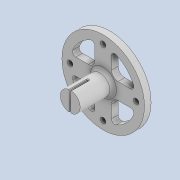
# Autodesk Inventor part: tendon_wh_1_mod
Saved by Autodesk Inventor 2020 (Build 240168000, 168)
## iProperties
Created: 2020-12-06
Part Number: tendon_wh_1_mod
Material: Generic
Document SubType Name: Modeling
Designer: Shuang Peng
Density: 1 g/cm^3
Appearance: Default
Author: Shuang Peng
Autodesk Inventor part; units mm, degrees
ref_plane "YZ Plane" through (0, 0, 0) normal (1, 0, 0) x (0, 1, 0)
ref_plane "XZ Plane" through (0, 0, 0) normal (0, 1, 0) x (-1, 0, 0)
ref_plane "XY Plane" through (0, 0, 0) normal (0, 0, 1) x (1, 0, 0)
sketch "Sketch1" plane through (0, 0, 0) normal (0, 0, 1) x (1, 0, 0)
  circle A0 centre (-10, 0) radius 1 projected
  circle A1 centre (0, 10) radius 1 projected
  circle A2 centre (0, -10) radius 1 projected
  circle A3 centre (10, 0) radius 1 projected
  circle A4 centre (0, 0) radius 1.5 projected
  arc A5 (10.8355, 3.8525) -> (3.8525, 10.8355) centre (0, 0) ccw projected
  arc A6 (9.4222, 1.85) -> (10.8355, 3.8525) centre (9.4222, 3.35) ccw projected
  line L0 (9.4222, 1.85) -> (3.35, 1.85) projected
  arc A7 (1.85, 3.35) -> (3.35, 1.85) centre (3.35, 3.35) ccw projected
  line L1 (1.85, 3.35) -> (1.85, 9.4222) projected
  arc A8 (3.8525, 10.8355) -> (1.85, 9.4222) centre (3.35, 9.4222) ccw projected
  line L2 (-1.85, 9.4222) -> (-1.85, 3.35) projected
  arc A9 (-3.35, 1.85) -> (-1.85, 3.35) centre (-3.35, 3.35) ccw projected
  line L3 (-3.35, 1.85) -> (-9.4222, 1.85) projected
  arc A10 (-10.8355, 3.8525) -> (-9.4222, 1.85) centre (-9.4222, 3.35) ccw projected
  arc A11 (-3.8525, 10.8355) -> (-10.8355, 3.8525) centre (0, 0) ccw projected
  arc A12 (-1.85, 9.4222) -> (-3.8525, 10.8355) centre (-3.35, 9.4222) ccw projected
  line L4 (3.35, -1.85) -> (9.4222, -1.85) projected
  arc A13 (10.8355, -3.8525) -> (9.4222, -1.85) centre (9.4222, -3.35) ccw projected
  arc A14 (3.8525, -10.8355) -> (10.8355, -3.8525) centre (0, 0) ccw projected
  arc A15 (1.85, -9.4222) -> (3.8525, -10.8355) centre (3.35, -9.4222) ccw projected
  line L5 (1.85, -9.4222) -> (1.85, -3.35) projected
  arc A16 (3.35, -1.85) -> (1.85, -3.35) centre (3.35, -3.35) ccw projected
  line L6 (-1.85, -3.35) -> (-1.85, -9.4222) projected
  arc A17 (-3.8525, -10.8355) -> (-1.85, -9.4222) centre (-3.35, -9.4222) ccw projected
  arc A18 (-10.8355, -3.8525) -> (-3.8525, -10.8355) centre (0, 0) ccw projected
  arc A19 (-9.4222, -1.85) -> (-10.8355, -3.8525) centre (-9.4222, -3.35) ccw projected
  line L7 (-9.4222, -1.85) -> (-3.35, -1.85) projected
  arc A20 (-1.85, -3.35) -> (-3.35, -1.85) centre (-3.35, -3.35) ccw projected
  circle A21 centre (0, 0) radius 12.55 projected
  line L8 (0, -10) -> (0, 10) construction
  line L9 (2.5, -10) -> (2.5, 10)
  line L10 (-2.5, 10) -> (-2.5, -10)
  arc A22 (-2.5, -10) -> (2.5, -10) centre (0, -10) ccw
  arc A23 (2.5, 10) -> (-2.5, 10) centre (0, 10) ccw
  line L11 (10, 0) -> (-10, 0) construction
  line L12 (10, 2.5) -> (-10, 2.5)
  line L13 (-10, -2.5) -> (10, -2.5)
  arc A24 (10, -2.5) -> (10, 2.5) centre (10, 0) ccw
  arc A25 (-10, 2.5) -> (-10, -2.5) centre (-10, 0) ccw
  point P0 (0, 0)
  point P1 (0, 0)
  point P2 (0, 0)
  point P3 (-2.5, -2.5)
  point P4 (2.5, -2.5)
  point P5 (2.5, 2.5)
  point P6 (-2.5, 2.5)
  dimension "d0" = 5
  dimension "d1" = 5
  constraints: 16 end point, 8 point on circle, 8 tangent, 4 centre point, 2 midpoint, 2 parallel, 1 horizontal, 1 vertical
  measures "d0" diameter of A23
  measures "d1" diameter of A25
extrude "Extrusion1" add sketch "Sketch1" along normal blind 2 contours A0 | A1 | A2 | A3 | A4 | A24 A13 L4 A16 L9 A7 L0 A6 | A6 L0 A7 L9 L12 A24 | A23 L9 L12 A7 L1 A8 | A8 L1 A7 L12 A9 L2 A12 A23 | A24 L13 L9 A16 L4 A13 | A12 L2 A9 L12 L10 A23 | L9 A7 L12 | L9 A16 L13 A20 L10 A9 L12 A7 | L13 A16 L9 | L9 A22 A15 L5 A16 L13 | L12 A9 L10 | L10 A9 L3 A10 A25 L12 | A22 A17 L6 A20 L13 A16 L5 A15 | A10 L3 A9 L10 A20 L7 A19 A25 | A22 L10 L13 A20 L6 A17 | L13 L10 A20 | A19 L7 A20 L10 L13 A25
sketch "Sketch2" plane through (0, 0, 2) normal (0, 0, 1) x (1, 0, 0)
  line L0 (-2.5, -2.5) -> (-2.5, -10) projected
  arc A0 (-2.5, -10) -> (2.5, -10) centre (0, -10) ccw projected
  line L1 (2.5, -10) -> (2.5, -2.5) projected
  line L2 (2.5, -2.5) -> (10, -2.5) projected
  arc A1 (10, -2.5) -> (10, 2.5) centre (10, 0) ccw projected
  line L3 (10, 2.5) -> (2.5, 2.5) projected
  line L4 (2.5, 2.5) -> (2.5, 10) projected
  arc A2 (2.5, 10) -> (-2.5, 10) centre (0, 10) ccw projected
  line L5 (-2.5, 10) -> (-2.5, 2.5) projected
  line L6 (-2.5, 2.5) -> (-10, 2.5) projected
  arc A3 (-10, 2.5) -> (-10, -2.5) centre (-10, 0) ccw projected
  line L7 (-10, -2.5) -> (-2.5, -2.5) projected
  point P0 (0, 0)
hole "Hole1" at (0, -10, 2) at (10, 0, 2) at (0, 10, 2) at (-10, 0, 2) direction (0, 0, -1) diameter 1.65 depth 5
sketch "Sketch3" plane through (0, 0, 2) normal (0, 0, 1) x (1, 0, 0)
  circle A0 centre (0, 0) radius 3
  dimension "d11" = 6
  constraints: 1 centre point, 1 coincident
  measures "d11" diameter of A0
extrude "Extrusion2" add sketch "Sketch3" along normal blind 6
fillet "Fillet1" radius 2 4 edges at (2.5, -2.5, 1) (-2.5, -2.5, 1) (-2.5, 2.5, 1) (2.5, 2.5, 1)
fillet "Fillet2" radius 1 1 edges at (-3, 0, 2)
sketch "Sketch4" plane through (0, 0, 8) normal (0, 0, 1) x (1, 0, 0)
  circle A0 centre (0, 0) radius 1
  dimension "d16" = 2
  constraints: 1 centre point, 1 coincident
  measures "d16" diameter of A0
extrude "Extrusion3" cut sketch "Sketch4" against normal blind 12
sketch "Sketch5" plane through (0, 0, 2) normal (0, 0, 1) x (1, 0, 0)
  arc A0 (2.5, 10) -> (-2.5, 10) centre (0, 10) ccw projected
  line L0 (-2.5, 10) -> (-2.5, 4.5) projected
  arc A1 (-4.5, 2.5) -> (-2.5, 4.5) centre (-4.5, 4.5) ccw projected
  line L1 (-4.5, 2.5) -> (-10, 2.5) projected
  arc A2 (-10, 2.5) -> (-10, -2.5) centre (-10, 0) ccw projected
  line L2 (-10, -2.5) -> (-4.5, -2.5) projected
  arc A3 (-2.5, -4.5) -> (-4.5, -2.5) centre (-4.5, -4.5) ccw projected
  line L3 (-2.5, -4.5) -> (-2.5, -10) projected
  arc A4 (-2.5, -10) -> (2.5, -10) centre (0, -10) ccw projected
  line L4 (2.5, -10) -> (2.5, -4.5) projected
  arc A5 (4.5, -2.5) -> (2.5, -4.5) centre (4.5, -4.5) ccw projected
  line L5 (4.5, -2.5) -> (10, -2.5) projected
  arc A6 (10, -2.5) -> (10, 2.5) centre (10, 0) ccw projected
  line L6 (10, 2.5) -> (4.5, 2.5) projected
  arc A7 (2.5, 4.5) -> (4.5, 2.5) centre (4.5, 4.5) ccw projected
  line L7 (2.5, 4.5) -> (2.5, 10) projected
  circle A8 centre (-10, 0) radius 0.825 projected
  circle A9 centre (10, 0) radius 0.825 projected
  circle A10 centre (0, -10) radius 0.825 projected
  circle A11 centre (0, 10) radius 0.825 projected
  circle A12 centre (0, 0) radius 4 projected
  circle A13 centre (0, 0) radius 1 projected
  circle A14 centre (0, 0) radius 12.5
  circle A15 centre (0, 0) radius 10
  point P0 (-2.5, -9.6825)
  point P1 (-9.6825, -2.5)
  point P2 (-12.5, 0)
  point P3 (0, -12.5)
  dimension "d19" = 25
  dimension "d20" = 20
  constraints: 2 centre point, 2 coincident
  measures "d19" diameter of A14
  measures "d20" diameter of A15
extrude "Extrusion4" add sketch "Sketch5" against normal blind 2 contours A2 L2 A15 L3 A4 A14
pattern_circular "Circular Pattern1" count 4 over 360 about axis through (0, 0, 2) along (0, 0, 1) of "Extrusion4"
fillet "Fillet3" radius 1 8 edges at (-2.5, -9.6825, 1) (-9.6825, -2.5, 1) (-9.6825, 2.5, 1) (-2.5, 9.6825, 1) (2.5, 9.6825, 1) (9.6825, 2.5, 1) (9.6825, -2.5, 1) (2.5, -9.6825, 1)
sketch "Sketch6" plane through (0, 0, 8) normal (0, 0, 1) x (1, 0, 0)
  circle A0 centre (0, 0) radius 1 projected
  circle A1 centre (0, 0) radius 3 projected
extrude "Extrusion5" add sketch "Sketch6" against normal up to surface (8 mm away) contours A0
thicken "Thicken1" operation add thickness 4 both sides no extend neighbours yes toward (0, 0, 1) faces at (-0.5351, 1.0949, 8)
sketch "Sketch7" plane through (0, 0, 12) normal (0, 0, 1) x (1, 0, 0)
  circle A0 centre (0, 0) radius 3 projected
  line L0 (-0.2, 6) -> (0.2, 6)
  line L1 (0.2, 6) -> (0.2, -6)
  line L2 (0.2, -6) -> (-0.2, -6)
  line L3 (-0.2, -6) -> (-0.2, 6)
  line L4 (-0.2, 6) -> (0.2, -6) construction
  line L5 (0.2, 6) -> (-0.2, -6) construction
  point P0 (-0.2, 2.9933)
  point P1 (-0.2, -2.9933)
  point P2 (0.2, -2.9933)
  point P3 (0.2, 2.9933)
  dimension "d31" = 0.4
  dimension "d32" = 12
  constraints: 12 end point, 2 midpoint, 2 parallel, 1 horizontal, 1 perpendicular
  measures "d31" distance of L0.start L0.end
  measures "d32" distance of L0.end L1.end
extrude "Extrusion6" cut sketch "Sketch7" against normal blind 5.5 contours L1 A0 L3
fillet "Fillet4" radius 0.2 2 edges at (-0.2, 0, 6.5) (0.2, 0, 6.5)
chamfer "Chamfer1" distance 0.2 angle 45 10 edges at (-0.2, -2.9933, 9.35) (0, -3, 6.5) (-0.142, -2.9966, 6.5591) (0.142, -2.9966, 6.5591) (0.2, -2.9933, 9.35) (-0.2, 2.9933, 9.35) (-0.142, 2.9966, 6.5591) (0, 3, 6.5) (0.142, 2.9966, 6.5591) (0.2, 2.9933, 9.35)
body "Solid1"
